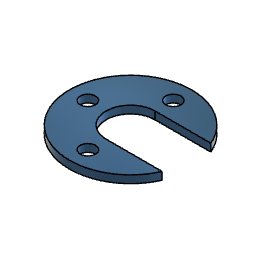
3d03 v1 (Autodesk Fusion 360 design; units mm, degrees)
Autodesk Fusion 360 part; units mm, degrees
sketch "Sketch1" plane through (0, 0, 0) normal (0, 1, 0) x (1, 0, 0)
  line L0 (0, 0) -> (0, 60) construction
  line L1 (0, 0) -> (0, -86.7996) construction
  line L2 (0, 0) -> (-80, 0) construction
  line L3 (0, 0) -> (75.5997, 0) construction
  circle A0 centre (0.0136, 28) radius 5
  circle A1 centre (-28, 0) radius 5
  circle A2 centre (0, -28) radius 5
  arc A3 (0, 16) -> (0, -16) centre (0, 0) ccw
  line L4 (0, 16) -> (36.6606, 16)
  line L5 (0, -16) -> (36.6606, -16)
  arc A4 (36.6606, 16) -> (36.6606, -16) centre (0, 0) ccw
  dimension "d1" = 80
  dimension "d2" = 10
  dimension "d3" = 10
  dimension "d4" = 10
  dimension "d5" = 28
  dimension "d6" = 28
  dimension "d7" = 28
  dimension "d8" = 32
  constraint coincident L0.start L1.start
  constraint vertical L0
  constraint parallel L0 L1
  constraint perpendicular L0 L2
  constraint perpendicular L1 L3
  constraint coincident L1 A2.centre
  constraint coincident L2 A1.centre
  constraint concentric A3 A4
  constraint coincident L0 A3.start
  constraint coincident L1 A3.end
  constraint perpendicular L0 L4
  constraint horizontal L5
  measures "d1" diameter of A4
  measures "d2" diameter of A0
  measures "d3" diameter of A1
  measures "d4" diameter of A2
  measures "d5" vertical distance of L0.start A0.centre
  measures "d6" vertical distance of L0.start A2.centre
  measures "d7" distance of L0.start A1.centre
  measures "d8" diameter of A3
extrude "Extrude1" add sketch "Sketch1" along normal blind 5
